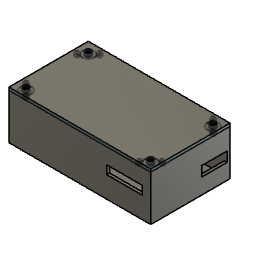
box_wemos (Autodesk Fusion 360 design; units mm, degrees)
Autodesk Fusion 360 part; units mm, degrees
note: some values were not read from the file. Set by a fixed rule: which face or edge a step refers to.
other "Base Mesh Feature1"
other "Scale1"
other "MeshRepair1"
other "MeshRepair2"
other "Modify1"
sketch "Sketch1" plane through (0, 0, 0) normal (0, 1, 0) x (1, 0, 0) in component "Box"
  line L0 (36, 26) -> (-60, 26)
  line L1 (-60, 26) -> (-60, -26)
  line L2 (-60, -26) -> (36, -26)
  line L3 (36, -26) -> (36, 26)
  line L4 (-60, 28) -> (38, 28)
  line L5 (38, 28) -> (38, -28)
  line L6 (38, -28) -> (-62, -28)
  line L7 (-62, -28) -> (-62, 28)
  line L8 (-62, 28) -> (-60, 28)
  circle A0 centre (9.7, 20.85) radius 1.85
  circle A1 centre (30.5, -21.05) radius 1.85
  circle A2 centre (-29.95, -20.95) radius 1.85
  circle A3 centre (-29.95, -20.95) radius 1.35
  circle A4 centre (30.5, -21.05) radius 1.35
  circle A5 centre (9.7, 20.85) radius 1.35
  circle A6 centre (9.7, 20.85) radius 2.5
  circle A7 centre (30.5, -21.05) radius 2.5
  circle A8 centre (-29.95, -20.95) radius 2.5
  line L9 (-11, 28) -> (-11, 38)
  line L10 (-6, 28) -> (-16, 28)
  line L11 (-16, 28) -> (-16, 38)
  line L12 (-16, 38) -> (-6, 38)
  line L13 (-6, 38) -> (-6, 28)
  line L14 (-6, 28) -> (-16, 38) construction
  line L15 (-16, 28) -> (-6, 38) construction
  line L16 (-4, 26) -> (-18, 26)
  line L17 (-18, 26) -> (-18, 40)
  line L18 (-18, 40) -> (-4, 40)
  line L19 (-4, 40) -> (-4, 26)
  line L20 (-4, 26) -> (-18, 40) construction
  line L21 (-18, 26) -> (-4, 40) construction
  line L22 (-18, 38) -> (-4, 38)
  line L23 (-23.2479, -11.5738) -> (-23.2479, 15.9262)
  line L24 (-23.2479, 15.9262) -> (-54.7479, 15.9262)
  circle A9 centre (-54.7479, 15.9262) radius 2
  circle A10 centre (-54.7479, 15.9262) radius 3.5
  line L25 (-54.7479, 19.4262) -> (-60, 19.4262)
  line L26 (-54.7479, 12.4262) -> (-60, 12.4262)
  point P0 (-11, 33)
  point P1 (-11, 33)
  dimension "d2" = 3.7
  dimension "d3" = 3.7
  dimension "d4" = 3.7
  dimension "d5" = 2.7
  dimension "d6" = 2.7
  dimension "d7" = 2.7
  dimension "d12" = 5
  dimension "d13" = 5
  dimension "d14" = 5
  dimension "d61" = 27.5
  dimension "d62" = 31.5
  dimension "d63" = 4
  dimension "d64" = 7
  constraint horizontal L0
  constraint vertical L1
  constraint horizontal L2
  constraint vertical L3
  constraint perpendicular L4 L5
  constraint perpendicular L5 L6
  constraint perpendicular L2 L7
  constraint perpendicular L7 L8
  constraint concentric A2 A3
  constraint concentric A1 A4
  constraint concentric A0 A5
  constraint concentric A0 A6
  constraint concentric A4 A7
  constraint concentric A3 A8
  constraint midpoint L4 L9.start
  constraint perpendicular L4 L9
  constraint horizontal L10
  constraint perpendicular L10 L11
  constraint parallel L10 L12
  constraint parallel L11 L13
  constraint coincident L14 P1
  constraint coincident L15 P1
  constraint coincident L4 L10.start
  constraint midpoint L9 P1
  constraint horizontal L16
  constraint perpendicular L16 L17
  constraint parallel L16 L18
  constraint parallel L17 L19
  constraint coincident L20 P1
  constraint coincident L21 P1
  constraint coincident L0 L16.start
  constraint coincident P1 P0
  constraint coincident L17 L22.start
  constraint coincident L19 L22.end
  constraint perpendicular L19 L22
  constraint parallel L1 L23
  constraint perpendicular L23 L24
  constraint coincident L24.end A9.centre
  constraint concentric A9 A10
  constraint coincident A10 L25.start
  constraint coincident L1 L25.end
  constraint tangent A10 L25
  constraint perpendicular L1 L25
  constraint coincident A10 L26.start
  constraint coincident L1 L26.end
  constraint tangent A10 L26
  constraint perpendicular L1 L26
  measures "d2" diameter of A0
  measures "d3" diameter of A1
  measures "d4" diameter of A2
  measures "d5" diameter of A3
  measures "d6" diameter of A4
  measures "d7" diameter of A5
  measures "d12" diameter of A6
  measures "d13" diameter of A7
  measures "d14" diameter of A8
  measures "d61" distance of L23.start L23.end
  measures "d62" distance of L23.end L24.end
  measures "d63" diameter of A9
  measures "d64" diameter of A10
extrude "Extrude1" add sketch "Sketch1" along normal blind 30 contours L0 L1 L2 L3 L4 L5 L6 L7 L8 L17 L19 | L0 L4 L10 L16 L17 L19 makes body 1 in component "Box"
extrude "Extrude2" add sketch "Sketch1" against normal blind 2 contours L0 L1 L2 L3 L16 A10 L25 L26 | L0 L1 L2 L3 L4 L5 L6 L7 L8 L17 L19 | L0 L4 L10 L16 L17 L19 | L1 A10 L25 L26 | A10 | A0 | A1 | A2 | A3 | A4 | A5 | A6 | A7 | A8 | A9 bodies 1 in component "Box"
extrude "Extrude3" add sketch "Sketch1" along normal blind 8 contours A0 | A1 | A2 bodies 1 in component "Box"
extrude "Extrude4" add sketch "Sketch1" along normal blind 5 contours A6 | A7 | A8 bodies 1 in component "Box"
extrude "Extrude5" add sketch "Sketch1" along normal blind 3 contours A3 | A4 | A5 bodies 1 in component "Box"
sketch "Sketch2" plane through (0, 30, 0) normal (0, 1, 0) x (-1, 0, 0) in component "Box"
  line L0 (-36, -26) -> (-36, 26)
  line L1 (-36, 26) -> (60, 26)
  line L2 (60, 26) -> (60, -26)
  line L3 (60, -26) -> (-36, -26)
  line L4 (62, -28) -> (62, 28)
  line L5 (62, 28) -> (-38, 28)
  line L6 (-38, 28) -> (-38, -28)
  line L7 (-38, -28) -> (62, -28)
  circle A0 centre (56, -22) radius 4
  circle A1 centre (56, 22) radius 4
  circle A2 centre (-32, 22) radius 4
  circle A3 centre (-32, -22) radius 4
  circle A4 centre (56, -22) radius 2.25
  circle A5 centre (-32, -22) radius 2.25
  circle A6 centre (-32, 22) radius 2.25
  circle A7 centre (56, 22) radius 2.25
  line L8 (56, -18) -> (60, -18)
  line L9 (52, -22) -> (52, -26)
  line L10 (56, 18) -> (60, 18)
  line L11 (52, 22) -> (52, 26)
  line L12 (-32, 18) -> (-36, 18)
  line L13 (-28, 22) -> (-28, 26)
  line L14 (-32, -18) -> (-36, -18)
  line L15 (-28, -22) -> (-28, -26)
  dimension "d21" = 4
  dimension "d22" = 4
  dimension "d23" = 4
  dimension "d24" = 4
  dimension "d25" = 4.5
  dimension "d26" = 4.5
  dimension "d27" = 4.5
  dimension "d28" = 4.5
  constraint tangent L2 A0
  constraint tangent L3 A0
  constraint tangent L1 A1
  constraint tangent L2 A1
  constraint tangent L1 A2
  constraint tangent L0 A2
  constraint tangent L0 A3
  constraint tangent L3 A3
  constraint concentric A0 A4
  constraint concentric A3 A5
  constraint concentric A2 A6
  constraint concentric A1 A7
  constraint coincident A0 L8.start
  constraint coincident L2 L8.end
  constraint tangent A0 L8
  constraint perpendicular L2 L8
  constraint coincident A0 L9.start
  constraint coincident L3 L9.end
  constraint tangent A0 L9
  constraint perpendicular L3 L9
  constraint coincident A1 L10.start
  constraint coincident L2 L10.end
  constraint tangent A1 L10
  constraint perpendicular L2 L10
  constraint coincident A1 L11.start
  constraint coincident L1 L11.end
  constraint tangent A1 L11
  constraint perpendicular L1 L11
  constraint coincident A2 L12.start
  constraint coincident L0 L12.end
  constraint tangent A2 L12
  constraint perpendicular L0 L12
  constraint coincident A2 L13.start
  constraint coincident L1 L13.end
  constraint tangent A2 L13
  constraint perpendicular L1 L13
  constraint coincident A3 L14.start
  constraint coincident L0 L14.end
  constraint tangent A3 L14
  constraint perpendicular L0 L14
  constraint coincident A3 L15.start
  constraint coincident L3 L15.end
  constraint tangent A3 L15
  constraint perpendicular L3 L15
  measures "d21" radius of A0
  measures "d22" radius of A1
  measures "d23" radius of A2
  measures "d24" radius of A3
  measures "d25" diameter of A4
  measures "d26" diameter of A5
  measures "d27" diameter of A6
  measures "d28" diameter of A7
extrude "Extrude6" add sketch "Sketch2" against normal blind 10 contours L0 A3 L14 | L0 A2 L12 | L0 L3 A3 | A3 | L0 L1 A2 | A2 | L3 A3 L15 | L1 A2 L13 | L3 A0 L9 | L1 A1 L11 | L2 L3 A0 | A0 | L1 L2 A1 | A1 | L2 A0 L8 | L2 A1 L10 | A4 | A5 | A6 | A7 bodies 1 in component "Box"
extrude "Extrude7" cut sketch "Sketch2" against normal blind 7 contours A4 | A5 | A6 | A7 bodies 1 in component "Box"
extrude "Extrude1'" add sketch "Sketch2" along normal blind 2 separate body contours L0 A3 L14 | L0 L1 L2 L3 A0 A1 A2 A3 L8 L9 L10 L11 L12 L13 L14 L15 | L0 A2 L12 | L0 L3 A3 | A3 | L0 L1 A2 | A2 | L3 A3 L15 | L1 A2 L13 | L3 A0 L9 | L1 A1 L11 | L2 L3 A0 | A0 | L1 L2 A1 | A1 | L2 A0 L8 | L2 A1 L10 | L4 L5 L6 L7 makes body 2 in component "cover"
sketch "Sketch3" plane through (38, 0, 0) normal (1, 0, 0) x (0, 0, -1) in component "Box"
  line L0 (28, -2) -> (28, 30)
  line L1 (28, 30) -> (-28, 30)
  line L2 (-28, 30) -> (-28, -2)
  line L3 (-28, -2) -> (28, -2)
  line L4 (8, 16) -> (26, 16)
  line L5 (26, 16) -> (26, 9)
  line L6 (26, 9) -> (8, 9)
  line L7 (8, 9) -> (8, 16)
  constraint horizontal L4
  constraint vertical L5
  constraint horizontal L6
  constraint vertical L7
other "Modify2"
extrude "Extrude8" cut sketch "Sketch3" against normal blind 2 contours L4 L5 L6 L7 bodies 1 in component "Box"
sketch "Sketch1 (2)" plane through (0, 0, 28) normal (0, 0, 1) x (1, 0, 0)
  line L0 (38, -2) -> (38, 30)
  line L1 (38, 30) -> (-62, 30)
  line L2 (-62, 30) -> (-62, -2)
  line L3 (-62, -2) -> (38, -2)
  line L4 (7, 19) -> (32, 19)
  line L5 (32, 19) -> (32, 13)
  line L6 (32, 13) -> (7, 13)
  line L7 (7, 13) -> (7, 19)
  constraint horizontal L4
  constraint vertical L5
  constraint horizontal L6
  constraint vertical L7
extrude "Extrude9" cut sketch "Sketch1 (2)" against normal blind 2 contours L4 L5 L6 L7 bodies 1 in component "Box"
extrude "Extrude10" add sketch "Sketch1" along normal blind 2 separate body contours L12 L17 L18 L19 L22 makes body 3 in component "Box"
extrude "Extrude11" add sketch "Sketch1" along normal blind 6 contours L4 L13 L19 L22 | L4 L11 L17 L22 bodies 1 3 in component "Box"
chamfer "Chamfer1" distance 10 distance2 4 2 edges at (-5, 6, -38) (-17, 6, -38) measured on face at (-4.6667, 6, -31.3333) measured on face at (-17.3333, 6, -34.6667) on bodies 1 in component "Box"
fillet "Fillet1" radius 2 2 edges at (-4, 1, -40) (-18, 1, -40) on bodies 1 in component "Box"
extrude "Extrude12" add 1 faces at (-12.6667, 0, -39.3333) along direction (0, -1, 0) blind 2 on bodies 1 bodies 1 in component "Box"
extrude "Extrude13" add sketch "Sketch2" against normal blind 2 separate body contours L0 A3 L14 | L0 L1 L2 L3 A0 A1 A2 A3 L8 L9 L10 L11 L12 L13 L14 L15 | L0 A2 L12 | L3 A3 L15 | L1 A2 L13 | L3 A0 L9 | L1 A1 L11 | L2 A0 L8 | L2 A1 L10 makes body 4 in component "Box"
copy_body "CutPasteBodies1" bodies 4 removing the originals makes body 5 in component "cover"
extrude "Extrude2'" cut 3 faces at (-53.3333, 29.3333, 26) (1.3333, 29.3333, 26) (30.6667, 29.3333, 26) along direction (0, 0, -1) blind 0.5 on bodies 5 bodies 5 in component "cover"
extrude "Extrude3'" cut 1 faces at (-26.6667, 28.6667, -26) along direction (0, 0, 1) blind 0.5 on bodies 5 bodies 5 in component "cover"
extrude "Extrude4'" cut 1 faces at (-60, 29.3333, 7.3333) along direction (1, 0, 0) blind 0.5 on bodies 5 bodies 5 in component "cover"
extrude "Extrude5'" cut 1 faces at (36, 29.3333, -7.3333) along direction (-1, 0, 0) blind 0.5 on bodies 5 bodies 5 in component "cover"
move_face "OffsetFaces1" offset -0.5 1 faces at (32.313, 29.3333, -18.0123) on bodies 5 in component "cover"
move_face "OffsetFaces2" offset -0.5 3 faces at (29.728, 29.3333, 25.2921) (-53.2422, 28.6667, -19.1026) (-59.2921, 29.3333, 19.728) on bodies 5 in component "cover"
combine "Combine1" operation add target body 2 tool bodies 5 in component "cover"
extrude "Extrude14" add sketch "Sketch1" along normal blind 16 contours A10 bodies 1 in component "Box"
extrude "Extrude15" add sketch "Sketch1" along normal blind 10 contours A9 bodies 1 in component "Box"
move_face "OffsetFaces3" offset 0.25 4 faces at (-58.2388, 30.6667, -22.224) (-56.6094, 31.3333, 24.1659) (33.571, 31.3333, 23.6107) (33.571, 31.3333, -20.3893) on bodies 2 in component "cover"
extrude "Extrude16" add sketch "Sketch1" along normal blind 16 contours L1 A10 L25 L26 bodies 1 in component "Box"
extrude "Extrude6'" cut sketch "Sketch2" against normal blind 2 contours L0 A3 L14 | L0 A2 L12 | L3 A3 L15 | L1 A2 L13 | L3 A0 L9 | L1 A1 L11 | L2 A0 L8 | L2 A1 L10 bodies 2 in component "cover"
component "Box" placed x (1, 0, 0) y (0, 1, 0) z (0, 0, 1) at (0, 0, 0)
component "cover" placed x (1, 0, 0) y (0, 1, 0) z (0, 0, 1) at (0, 0, 0)
named bodies: "box_box", "box_cover"
